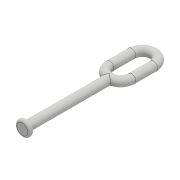
# Autodesk Inventor part: Elo-Bola Longo
Saved by Autodesk Inventor 2018 (Build 220112000, 112)
## iProperties
Created: 2021-04-27
Part Number: Elo-Bola Longo
Material: Generic
Document SubType Name: Modeling
Designer: l01767
Density: 1 g/cm^3
Appearance: Default
Author: l01767
Autodesk Inventor part; units mm, degrees
ref_plane "YZ Plane" through (0, 0, 0) normal (1, 0, 0) x (0, 1, 0)
ref_plane "XZ Plane" through (0, 0, 0) normal (0, 1, 0) x (-1, 0, 0)
ref_plane "XY Plane" through (0, 0, 0) normal (0, 0, 1) x (1, 0, 0)
sketch "Sketch1" plane through (0, 0, 0) normal (0, 0, 1) x (1, 0, 0)
  line L0 (0, 0) -> (0, 195)
  line L1 (0, 195) -> (0, 295) construction
  line L2 (25, 220) -> (25, 270)
  line L3 (-25, 270) -> (-25, 220)
  arc A0 (-25, 220) -> (25, 220) centre (0, 220) ccw
  arc A1 (25, 270) -> (-25, 270) centre (0, 270) ccw
  point P0 (0, 245)
  dimension "d0" = 195
  dimension "d1" = 100
  dimension "d2" = 50
  constraints: 10 end point, 6 point on circle, 4 tangent, 2 centre point, 2 point on line, 2 vertical, 1 midpoint, 1 parallel
  measures "d0" distance of L0.start L0.end
  measures "d1" distance of L0.end L1.end
  measures "d2" diameter of A1
sketch "Sketch2" plane through (0, 0, 0) normal (0, 1, 0) x (-1, 0, 0)
  circle A0 centre (0, 0) radius 10
  dimension "d3" = 20
  constraints: 1 centre point, 1 coincident
  measures "d3" diameter of A0
sweep "Sweep1" add profiles "Sketch2" path "Sketch1" path curves L0
sketch "Sketch3" plane through (0, 0, 0) normal (1, 0, 0) x (0, 1, 0)
  line L0 (195, -10) -> (195, 10) projected
  circle A0 centre (195, 0) radius 10
  point P0 (0, 0)
  dimension "d6" = 20
  constraints: 1 centre point, 1 midpoint
  measures "d6" diameter of A0
sweep "Sweep2" add profiles "Sketch3" path "Sketch1" path curves A0 L3 A1 L2
sketch "Sketch4" plane through (0, 0, 0) normal (1, 0, 0) x (0, 1, 0)
  line L0 (0, 12.5) -> (0, -12.5) construction
  line L1 (5, 12.5) -> (5, -12.5)
  line L2 (-5, -12.5) -> (-5, 12.5)
  arc A0 (5, 12.5) -> (-5, 12.5) centre (0, 12.5) ccw
  arc A1 (-5, -12.5) -> (5, -12.5) centre (0, -12.5) ccw
  line L3 (-5, 0) -> (5, 0)
  point P0 (0, 0)
  dimension "d9" = 25
  dimension "d10" = 5
  constraints: 10 end point, 4 point on circle, 4 tangent, 3 midpoint, 2 centre point, 1 parallel, 1 vertical
  measures "d9" distance of L0.start L0.end
  measures "d10" radius of A1
revolve "Revolution1" add sketch "Sketch4" angle 360 about axis through (0, -5, 0) along (0, 1, 0) contours L1 L3 L2 A0
body "Solid1"
